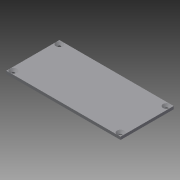
# Autodesk Inventor part: case cover
Saved by Autodesk Inventor 2015 (Build 190159000, 159)
## iProperties
Created: 2019-05-19
Part Number: case cover
Material: Generic
Document SubType Name: Modeling
Designer: Toby
Density: 1 g/cm^3
Appearance: Default
Author: Toby
Autodesk Inventor part; units mm, degrees
ref_plane "YZ Plane" through (0, 0, 0) normal (1, 0, 0) x (0, 1, 0)
ref_plane "XZ Plane" through (0, 0, 0) normal (0, 1, 0) x (-1, 0, 0)
ref_plane "XY Plane" through (0, 0, 0) normal (0, 0, 1) x (1, 0, 0)
sketch "Sketch1" plane through (0, 0, 0) normal (0, 0, 1) x (1, 0, 0)
  line L0 (-46.9696, 22.7927) -> (33.4304, 22.7927)
  line L1 (33.4304, 22.7927) -> (33.4304, -14.6073)
  line L2 (33.4304, -14.6073) -> (-46.9696, -14.6073)
  line L3 (-46.9696, -14.6073) -> (-46.9696, 22.7927)
  circle A0 centre (-44.4696, 20.2927) radius 1
  circle A1 centre (-44.4696, -12.1073) radius 1
  circle A2 centre (30.9304, -12.1073) radius 1
  circle A3 centre (30.9304, 20.2927) radius 1
  point P0 (0, 0)
  dimension "d0" = 80.4
  dimension "d1" = 37.4
  dimension "d2" = 75.4
  dimension "d3" = 32.4
  dimension "d4" = 32.4
  dimension "d5" = 75.4
  dimension "d6" = 2.5
  dimension "d7" = 2.5
  dimension "d8" = 2
  dimension "d9" = 2
  dimension "d10" = 2
  dimension "d11" = 2
  constraints: 8 end point, 4 centre point, 4 coincident, 2 parallel, 1 horizontal, 1 perpendicular
  measures "d0" distance of L0.start L0.end
  measures "d1" distance of L2.end L0.start
  measures "d2" distance of point (30.93, 20.293) point (-44.47, 20.293)
  measures "d3" distance of point (-44.47, -12.107) point (-44.47, 20.293)
  measures "d4" distance of point (30.93, -12.107) point (30.93, 20.293)
  measures "d5" distance of point (-44.47, -12.107) point (30.93, -12.107)
  measures "d6" distance from line of L0 point (30.93, 20.293)
  measures "d7" distance from line of L1 point (30.93, 20.293)
  measures "d8" diameter of A0
  measures "d9" diameter of A1
  measures "d10" diameter of A2
  measures "d11" diameter of A3
extrude "Extrusion1" add sketch "Sketch1" along normal blind 2
sketch "Sketch2" plane through (0, 0, 2) normal (0, 0, 1) x (1, 0, 0)
  circle A0 centre (-44.4696, 20.2927) radius 1 projected
  circle A1 centre (-44.4696, -12.1073) radius 1 projected
  circle A2 centre (30.9304, -12.1073) radius 1 projected
  circle A3 centre (30.9304, 20.2927) radius 1 projected
  point P0 (0, 0)
  constraints: 4 coincident
hole "Hole1" at (-44.4696, 20.2927, 2) at (-44.4696, -12.1073, 2) at (30.9304, -12.1073, 2) at (30.9304, 20.2927, 2) direction (0, 0, -1) diameter 2 depth 8 tip angle 118 countersink diameter 5 countersink angle 90
body "Solid1"
